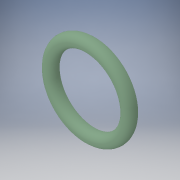
# Autodesk Inventor part: joint
Saved by Autodesk Inventor 2019 (Build 230136000, 136)
## iProperties
Created: 2018-04-27
Part Number: joint
Material: Caoutchouc, silicone
Document SubType Name: Modeling
Designer: Theo
Density: 1.25 g/cm^3
Appearance: Caoutchouc - Vert
Author: Theo
Autodesk Inventor part; units mm, degrees
ref_plane "YZ Plane" through (0, 0, 0) normal (1, 0, 0) x (0, 1, 0)
ref_plane "XZ Plane" through (0, 0, 0) normal (0, 1, 0) x (-1, 0, 0)
ref_plane "XY Plane" through (0, 0, 0) normal (0, 0, 1) x (1, 0, 0)
sketch "Esquisse1" plane through (0, 0, 0) normal (1, 0, 0) x (0, 1, 0)
  circle A0 centre (12.5, 0) radius 2
  line L0 (10.5, 2) -> (10.5, -2) construction
  line L1 (0, 14.3564) -> (0, -27.2029)
  point P0 (0, 0)
  dimension "d0" = 4
  dimension "d2" = 21
  constraints: 4 end point, 2 vertical, 1 centre point, 1 horizontal alignment, 1 point on line, 1 tangent
  measures "d0" diameter of A0
  measures "d2" diameter of L0 L1
revolve "Révolution1" add sketch "Esquisse1" angle 360 about axis through (0, 0, 14.3564) along (0, 0, -1)
equation "\"d2\" = d175"
equation "\"d175\" = 21"
